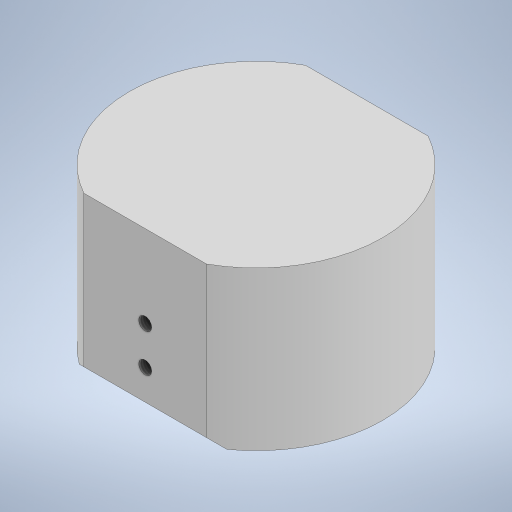
# Autodesk Inventor part: BaseSupport
Saved by Autodesk Inventor 2023 (Build 270158000, 158)
## iProperties
Created: 2023-02-24
Part Number: BaseSupport
Material: Generic
Document SubType Name: Modeling
Designer: roota
Density: 1 g/cm^3
Appearance: Default
Author: roota
Autodesk Inventor part; units mm, degrees
ref_plane "YZ Plane" through (0, 0, 0) normal (1, 0, 0) x (0, 1, 0)
ref_plane "XZ Plane" through (0, 0, 0) normal (0, 1, 0) x (-1, 0, 0)
ref_plane "XY Plane" through (0, 0, 0) normal (0, 0, 1) x (1, 0, 0)
sketch "Sketch1" plane through (0, 0, 0) normal (0, 1, 0) x (-1, 0, 0)
  circle A0 centre (0, 0) radius 70 construction
  line L0 (32.2622, 28.3815) -> (0.4069, 28.3815) construction
  line L1 (0.4069, 28.3815) -> (0.4069, 1.4276) construction
  line L2 (0.4069, 1.4276) -> (32.2622, 1.4276) construction
  line L3 (32.2622, 1.4276) -> (32.2622, 28.3815) construction
  line L4 (21.4142, 1.4276) -> (78.1619, 1.4276) construction
  line L5 (78.1619, 1.4276) -> (78.1619, -1.5168) construction
  line L6 (78.1619, -1.5168) -> (21.4142, -1.5168) construction
  line L7 (21.4142, -1.5168) -> (21.4142, 1.4276) construction
  line L8 (8.448, -42.1306) -> (24.3757, -14.5431) construction
  line L9 (24.3757, -14.5431) -> (1.0329, -1.0662) construction
  line L10 (1.0329, -1.0662) -> (-14.8947, -28.6537) construction
  line L11 (-14.8947, -28.6537) -> (8.448, -42.1306) construction
  line L12 (-9.4708, -19.2591) -> (-37.8446, -68.404) construction
  line L13 (-37.8446, -68.404) -> (-40.3946, -66.9318) construction
  line L14 (-40.3946, -66.9318) -> (-12.0207, -17.7868) construction
  line L15 (-12.0207, -17.7868) -> (-9.4708, -19.2591) construction
  line L16 (-40.7102, 13.7491) -> (-24.7826, -13.8384) construction
  line L17 (-24.7826, -13.8384) -> (-1.4398, -0.3614) construction
  line L18 (-1.4398, -0.3614) -> (-17.3674, 27.2261) construction
  line L19 (-17.3674, 27.2261) -> (-40.7102, 13.7491) construction
  line L20 (-11.9435, 17.8314) -> (-40.3173, 66.9764) construction
  line L21 (-40.3173, 66.9764) -> (-37.7673, 68.4486) construction
  line L22 (-37.7673, 68.4486) -> (-9.3935, 19.3037) construction
  line L23 (-9.3935, 19.3037) -> (-11.9435, 17.8314) construction
  circle A1 centre (0, 0) radius 40
  dimension "d0" = 140
  dimension "d3" = 360
  dimension "d5" = 80
  constraints: 48 end point, 6 coincident, 4 parallel, 3 point on line, 2 centre point, 2 horizontal, 2 perpendicular, 53 other
  measures "d0" diameter of A0
  measures "d5" diameter of A1
extrude "Extrusion1" add sketch "Sketch1" along normal blind 50
sketch "Sketch2" plane through (0, 50, 0) normal (0, 1, 0) x (1, 0, 0)
  circle A0 centre (0, 0) radius 40 projected
  line L0 (-19.3649, -35) -> (19.3649, -35)
  line L1 (-19.3649, 35) -> (19.3649, 35)
  point P0 (0, -35)
  dimension "d8" = 70
  constraints: 4 end point, 4 point on circle, 2 parallel, 1 horizontal, 1 midpoint
  measures "d8" distance from line of point (0, -35) L1
extrude "Extrusion2" cut sketch "Sketch2" against normal blind 60 contours L1 A0 | A0 L0
sketch "Sketch3" plane through (-19.3649, 50, 35) normal (0, 0, 1) x (1, 0, 0)
  line L0 (38.7298, -50) -> (0, -50) projected
  point P0 (19.3649, -50)
  point P1 (19.3649, -38)
  point P2 (19.3649, -50)
  point P3 (19.3649, -26)
  point P4 (19.3649, -50)
  dimension "d11" = 12
  dimension "d12" = 12
  constraints: 2 midpoint, 2 vertical alignment
  measures "d11" distance of point (19.365, -50) point (19.365, -38)
  measures "d12" distance of point (19.365, -38) point (19.365, -26)
hole "Hole1" at (0, 12, 35) at (0, 24, 35) direction (0, 0, -1) diameter 4.134 depth 15 tip angle 118 thread size "M5x0.8" class "6H" standard "ISO Metric profile"
mirror "Mirror1" about plane through (0, 0, 0) normal (0, 0, 1) of "Hole1"
chamfer "Chamfer1" distance 2.5 angle 45 2 edges at (0, 0, 35) (0, 0, -35)
body "Solid1"
